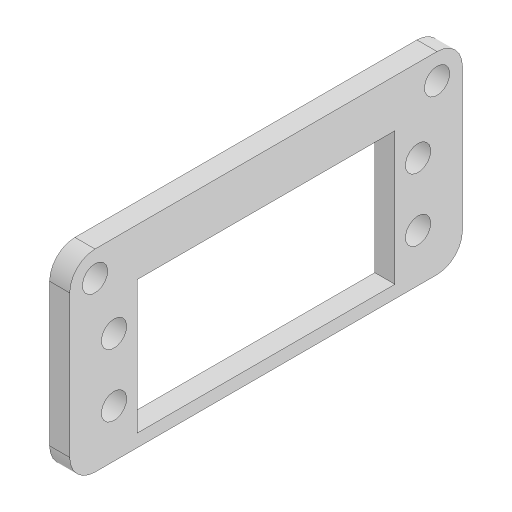
# Autodesk Inventor part: servoPlate
Saved by Autodesk Inventor 2023 (Build 270158000, 158)
## iProperties
Created: 2022-09-10
Part Number: servoPlate
Material: Generic
Document SubType Name: Modeling
Designer: deli
Density: 1 g/cm^3
Appearance: Default
Author: deli
Autodesk Inventor part; units mm, degrees
ref_plane "YZ Plane" through (0, 0, 0) normal (1, 0, 0) x (0, 1, 0)
ref_plane "XZ Plane" through (0, 0, 0) normal (0, 1, 0) x (-1, 0, 0)
ref_plane "XY Plane" through (0, 0, 0) normal (0, 0, 1) x (1, 0, 0)
sketch "Sketch1" plane through (0, 0, 0) normal (1, 0, 0) x (0, 1, 0)
  circle A0 centre (109.1688, 245.7866) radius 2
  circle A1 centre (109.1688, 197.7866) radius 2
  circle A2 centre (99.2688, 197.7866) radius 2
  circle A3 centre (99.2688, 245.7866) radius 2
  line L0 (109.1688, 245.7866) -> (109.1688, 197.7866) construction
  line L1 (109.1688, 197.7866) -> (99.2688, 197.7866) construction
  line L2 (99.2688, 197.7866) -> (99.2688, 245.7866) construction
  line L3 (99.2688, 245.7866) -> (109.1688, 245.7866) construction
  line L4 (114.2188, 248.9366) -> (94.2188, 248.9366) construction
  line L5 (94.2188, 248.9366) -> (94.2188, 194.6366) construction
  line L6 (94.2188, 194.6366) -> (114.2188, 194.6366) construction
  line L7 (114.2188, 194.6366) -> (114.2188, 248.9366) construction
  line L8 (114.2188, 241.6366) -> (94.2188, 241.6366) construction
  line L9 (94.2188, 241.6366) -> (94.2188, 201.9366) construction
  line L10 (94.2188, 201.9366) -> (114.2188, 201.9366) construction
  line L11 (114.2188, 201.9366) -> (114.2188, 241.6366) construction
  line L12 (93.7188, 242.1366) -> (114.7188, 242.1366)
  line L13 (114.7188, 242.1366) -> (114.7188, 201.4366)
  line L14 (114.7188, 201.4366) -> (93.7188, 201.4366)
  line L15 (93.7188, 201.4366) -> (93.7188, 242.1366)
  circle A4 centre (118.2188, 248.7866) radius 2
  circle A5 centre (118.2188, 194.7866) radius 2
  arc A6 (122.2188, 248.7866) -> (118.2188, 252.7866) centre (118.2188, 248.7866) ccw
  arc A7 (118.2188, 190.7866) -> (122.2188, 194.7866) centre (118.2188, 194.7866) ccw
  arc A8 (91.7188, 194.7866) -> (95.7188, 190.7866) centre (95.7188, 194.7866) ccw
  arc A9 (95.7188, 252.7866) -> (91.7188, 248.7866) centre (95.7188, 248.7866) ccw
  line L16 (122.2188, 248.1479) -> (122.2188, 194.1479) construction
  line L17 (118.2188, 190.7866) -> (95.7188, 190.7866)
  line L18 (91.7188, 194.7866) -> (91.7188, 248.7866)
  line L19 (95.7188, 252.7866) -> (118.2188, 252.7866)
  line L20 (122.2188, 248.7866) -> (122.2188, 194.7866)
  point P0 (0, 0)
  dimension "d0" = 4
  dimension "d1" = 4
  dimension "d2" = 4
  dimension "d3" = 4
  dimension "d4" = 9.9
  dimension "d5" = 48
  dimension "d7" = 20
  dimension "d8" = 5.05
  dimension "d9" = 3.15
  dimension "d10" = 39.7
  dimension "d11" = 7.3
  dimension "d12" = 0.5
  dimension "d14" = 4
  dimension "d16" = 4
  dimension "d18" = 2
  dimension "d20" = 2
  dimension "d28" = 54
  dimension "d30" = 2
  dimension "d31" = 7.5
  dimension "d32" = 62
  dimension "d33" = 3.85
  dimension "d34" = 54.3
  dimension "d40" = 54
  constraints: 42 end point, 10 centre point, 10 tangent, 9 perpendicular, 8 point on circle, 6 parallel, 2 coincident, 2 horizontal, 2 point on line, 2 vertical, 3 other
  measures "d0" diameter of A0
  measures "d1" diameter of A3
  measures "d2" diameter of A1
  measures "d3" diameter of A2
  measures "d4" distance of L2.end L0.start
  measures "d5" distance of L0.start L0.end
  measures "d7" distance of L5.end L6.end
  measures "d8" distance between parallel lines of L0 L7
  measures "d9" distance between parallel lines of L6 L1
  measures "d10" distance of L10.end L8.start
  measures "d11" distance between parallel lines of L6 L10
  measures "d12" distance between parallel lines of L8 L12
  measures "d14" diameter of A4
  measures "d16" diameter of A5
  measures "d18" radial gap between concentric circles of A6 A4
  measures "d20" radial gap between concentric circles of A5 A7
  measures "d28" distance of L16.start L16.end
  measures "d30" distance between parallel lines of L15 L18
  measures "d31" distance between parallel lines of L16 L13
  measures "d32" distance between parallel lines of L17 L19
  measures "d33" distance between parallel lines of L19 L4
  measures "d34" distance of L6.end L4.start
  measures "d40" distance of A5.centre A4.centre
extrude "Extrusion2" add sketch "Sketch1" along normal blind 3.175
equation "\"d1\" = d0"
equation "\"d2\" = d0"
equation "\"d3\" = d0"
equation "\"d8\" = -0.5 * d4 + 0.5 * d7"
equation "\"d9\" = -0.5 * d5 + 0.5 * d6"
equation "\"d11\" = -0.5 * d10 + 0.5 * d6"
equation "\"d14\" = d13"
equation "\"d16\" = d13"
equation "\"d18\" = d17"
equation "\"d20\" = d17"
equation "\"d33\" = -0.5 * d34 + 0.5 * d32"
equation "\"d40\" = d28"
equation "\"d6\" = 54.3"
equation "\"d13\" = 4"
equation "\"d17\" = 2"
body "Solid2"
